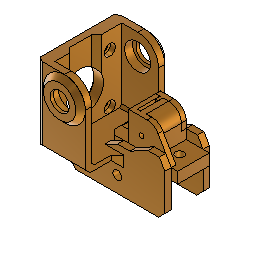
Worm Gear Buddy 0.8M Wide (Autodesk Fusion 360 design; units mm, degrees)
description: Worm Gear Drive bracket
part number: Worm Gear Buddy
Autodesk Fusion 360 part; units mm, degrees
note: some values were not read from the file. Chosen so that the rebuilt part matches the saved one: which face or edge a step refers to. Set by a fixed rule: which sketch regions a step uses; the direction of a hole.
sketch "Sketch2" plane through (0, 0, 0) normal (1, 0, 0) x (0, 1, 0)
  line L0 (0, 0) -> (48.25, 0)
  line L1 (50, 20) -> (50, 73.5)
  line L2 (0, 73.5) -> (0, 0)
  circle A0 centre (23, 42) radius 11.5
  line L3 (23, 0) -> (23, 73.5) construction
  line L4 (4, 73.5) -> (4, 23)
  line L5 (46, 73.5) -> (46, 23)
  line L6 (0, 20) -> (50, 20)
  line L7 (4, 23) -> (46, 23)
  line L8 (24.25, 20) -> (24.25, 0)
  line L9 (20.25, 20) -> (20.25, 0)
  line L10 (38.5, 26.5) -> (7.5, 26.5) construction
  line L11 (7.5, 26.5) -> (7.5, 57.5) construction
  line L12 (7.5, 57.5) -> (38.5, 57.5) construction
  line L13 (38.5, 57.5) -> (38.5, 26.5) construction
  line L14 (38.5, 26.5) -> (7.5, 57.5) construction
  line L15 (7.5, 26.5) -> (38.5, 57.5) construction
  line L16 (44.25, 20) -> (44.25, 0)
  line L17 (0, 73.5) -> (50, 73.5)
  line L18 (4, 20) -> (4, 0)
  circle A1 centre (7.5, 57.5) radius 3.5 construction
  line L19 (48.25, 20) -> (48.25, 0)
  dimension "d2076" = 0
  dimension "d2077" = 0
  dimension "d2078" = 0
  dimension "d2079" = 0
  dimension "d2092" = 0
  dimension "d2093" = 0
  dimension "d2094" = 0
  dimension "d2095" = 0
  dimension "d2312" = 0
  dimension "d2313" = 0
  dimension "d2314" = 0
  dimension "d2315" = 0
  dimension "d2324" = 0
  dimension "d2325" = 0
  dimension "d2326" = 0
  dimension "d2327" = 0
  dimension "d2544" = 0
  dimension "d2545" = 0
  dimension "d2546" = 0
  dimension "d2547" = 0
  dimension "d2572" = 0
  dimension "d2573" = 0
  dimension "d2574" = 0
  dimension "d2575" = 0
  dimension "d2728" = 0
  dimension "d2729" = 0
  dimension "d2730" = 0
  dimension "d2731" = 0
  dimension "d2896" = 0
  dimension "d2897" = 0
  dimension "d2898" = 0
  dimension "d2899" = 0
  dimension "d2949" = 0
  dimension "d2950" = 0
  dimension "d2951" = 0
  dimension "d2952" = 0
  dimension "d2957" = 0
  dimension "d2958" = 0
  dimension "d2959" = 0
  dimension "d2960" = 0
  dimension "d2961" = 0
  dimension "d2962" = 0
  dimension "d2963" = 0
  dimension "d2964" = 0
  dimension "d3029" = 0
  dimension "d3030" = 0
  dimension "d3031" = 0
  dimension "d3032" = 0
  dimension "d3037" = 0
  dimension "d3038" = 0
  dimension "d3039" = 0
  dimension "d3040" = 0
  dimension "d3045" = 0
  dimension "d3046" = 0
  dimension "d3047" = 0
  dimension "d3048" = 0
  dimension "d12_1" = 23
  dimension "d43" = 0
  dimension "d44" = 0
  dimension "d45" = 0
  dimension "d46" = 0
  dimension "d65" = 0
  dimension "d66" = 0
  dimension "d67" = 0
  dimension "d68" = 0
  dimension "d81" = 0
  dimension "d82" = 0
  dimension "d83" = 0
  dimension "d84" = 0
  dimension "d103" = 31.5
  dimension "d106" = 4
  dimension "d137" = 0
  dimension "d138" = 0
  dimension "d139" = 0
  dimension "d140" = 0
  dimension "d145" = 0
  dimension "d146" = 0
  dimension "d147" = 0
  dimension "d148" = 0
  dimension "d153" = 0
  dimension "d154" = 0
  dimension "d155" = 0
  dimension "d156" = 0
  dimension "d160" = 20
  dimension "d164" = 23
  dimension "d174" = 0
  dimension "d175" = 0
  dimension "d176" = 0
  dimension "d177" = 0
  dimension "d182" = 0
  dimension "d183" = 0
  dimension "d184" = 0
  dimension "d185" = 0
  dimension "d194" = 0
  dimension "d195" = 0
  dimension "d196" = 0
  dimension "d197" = 0
  dimension "d202" = 0
  dimension "d203" = 0
  dimension "d204" = 0
  dimension "d205" = 0
  dimension "d220" = 0
  dimension "d221" = 0
  dimension "d222" = 0
  dimension "d223" = 0
  dimension "d228" = 0
  dimension "d229" = 0
  dimension "d230" = 0
  dimension "d231" = 0
  dimension "d250" = 0
  dimension "d251" = 0
  dimension "d252" = 0
  dimension "d253" = 0
  dimension "d264" = 0
  dimension "d265" = 0
  dimension "d266" = 0
  dimension "d267" = 0
  dimension "d272" = 0
  dimension "d273" = 0
  dimension "d274" = 0
  dimension "d275" = 0
  dimension "d304" = 0
  dimension "d305" = 0
  dimension "d306" = 0
  dimension "d307" = 0
  dimension "d316" = 0
  dimension "d317" = 0
  dimension "d318" = 0
  dimension "d319" = 0
  dimension "d328" = 0
  dimension "d329" = 0
  dimension "d330" = 0
  dimension "d331" = 0
  dimension "d336" = 0
  dimension "d337" = 0
  dimension "d338" = 0
  dimension "d339" = 0
  dimension "d376" = 0
  dimension "d377" = 0
  dimension "d378" = 0
  dimension "d379" = 0
  dimension "d398" = 0
  dimension "d399" = 0
  dimension "d400" = 0
  dimension "d401" = 0
  dimension "d406" = 0
  dimension "d407" = 0
  dimension "d408" = 0
  dimension "d409" = 0
  dimension "d414" = 0
  dimension "d415" = 0
  dimension "d416" = 0
  dimension "d417" = 0
  dimension "d434" = 0
  dimension "d435" = 0
  dimension "d436" = 0
  dimension "d437" = 0
  dimension "d450" = 0
  dimension "d451" = 0
  dimension "d452" = 0
  dimension "d453" = 0
  dimension "d482" = 0
  dimension "d483" = 0
  dimension "d484" = 0
  dimension "d485" = 0
  dimension "d490" = 0
  dimension "d491" = 0
  dimension "d492" = 0
  dimension "d493" = 0
  dimension "d498" = 0
  dimension "d499" = 0
  dimension "d500" = 0
  dimension "d501" = 0
  dimension "d518" = 0
  dimension "d519" = 0
  dimension "d520" = 0
  dimension "d521" = 0
  dimension "d538" = 0
  dimension "d539" = 0
  dimension "d540" = 0
  dimension "d541" = 0
  dimension "d546" = 0
  dimension "d547" = 0
  dimension "d548" = 0
  dimension "d549" = 0
  dimension "d554" = 0
  dimension "d555" = 0
  dimension "d556" = 0
  dimension "d557" = 0
  dimension "d562" = 0
  dimension "d563" = 0
  dimension "d564" = 0
  dimension "d565" = 0
  dimension "d575" = 0
  dimension "d576" = 0
  dimension "d577" = 0
  dimension "d578" = 0
  dimension "d583" = 0
  dimension "d584" = 0
  dimension "d585" = 0
  dimension "d586" = 0
  dimension "d629" = 0
  dimension "d630" = 0
  dimension "d631" = 0
  dimension "d632" = 0
  dimension "d637" = 0
  dimension "d638" = 0
  dimension "d639" = 0
  dimension "d640" = 0
  dimension "d645" = 0
  dimension "d646" = 0
  dimension "d647" = 0
  dimension "d648" = 0
  dimension "d705" = 4
  dimension "d706" = 31
  dimension "d707" = 31
  dimension "d708" = 3
  dimension "d716" = 22
  dimension "d735" = 0
  dimension "d736" = 0
  dimension "d737" = 0
  dimension "d738" = 0
  dimension "d743" = 0
  dimension "d744" = 0
  dimension "d745" = 0
  dimension "d746" = 0
  dimension "d751" = 0
  dimension "d752" = 0
  dimension "d753" = 0
  dimension "d754" = 0
  dimension "d759" = 0
  dimension "d760" = 0
  dimension "d761" = 0
  dimension "d762" = 0
  dimension "d825" = 0
  dimension "d826" = 0
  dimension "d827" = 0
  dimension "d828" = 0
  dimension "d833" = 0
  dimension "d834" = 0
  dimension "d835" = 0
  dimension "d836" = 0
  dimension "d841" = 0
  dimension "d842" = 0
  dimension "d843" = 0
  dimension "d844" = 0
  dimension "d849" = 0
  dimension "d850" = 0
  dimension "d851" = 0
  dimension "d852" = 0
  dimension "d868" = 19
  dimension "d869" = 4
  dimension "d870" = 20
  dimension "d871" = 4
  dimension "d872" = 4
  dimension "d873" = 7
  dimension "d879" = 0
  dimension "d880" = 0
  dimension "d881" = 0
  dimension "d882" = 0
  dimension "d884" = 1.75
  dimension "d897" = 0
  dimension "d898" = 0
  dimension "d899" = 0
  dimension "d900" = 0
  dimension "d916" = 0
  dimension "d917" = 0
  dimension "d918" = 0
  dimension "d919" = 0
  dimension "d929" = 0
  dimension "d930" = 0
  dimension "d931" = 0
  dimension "d932" = 0
  dimension "d957" = 0
  dimension "d958" = 0
  dimension "d959" = 0
  dimension "d960" = 0
  dimension "d973" = 0
  dimension "d974" = 0
  dimension "d975" = 0
  dimension "d976" = 0
  dimension "d985" = 0
  dimension "d986" = 0
  dimension "d987" = 0
  dimension "d988" = 0
  dimension "d1013" = 0
  dimension "d1014" = 0
  dimension "d1015" = 0
  dimension "d1016" = 0
  dimension "d1021" = 0
  dimension "d1022" = 0
  dimension "d1023" = 0
  dimension "d1024" = 0
  dimension "d1029" = 0
  dimension "d1030" = 0
  dimension "d1031" = 0
  dimension "d1032" = 0
  dimension "d1037" = 0
  dimension "d1038" = 0
  dimension "d1039" = 0
  dimension "d1040" = 0
  measures "d12_1" diameter of A0
  measures "d706" distance of L0.start
  measures "d868" distance of L0.start
  measures "d872" distance of L0.start
  measures "d873" diameter of A1
extrude "Extrude1" add sketch "Sketch2" along normal blind 7 contours L1 L2 L4 L5 L6 L7 L17 | L4 L5 L7 L17 makes body 1
sketch "Sketch10" plane through (7, 0, 0) normal (1, 0, 0) x (0, 1, 0)
  line L0 (-7, 73.65) -> (7, 73.65)
  line L1 (7, 73.65) -> (7, 0)
  line L2 (7, 0) -> (-7, 0)
  line L3 (-7, 0) -> (-7, 73.65)
  circle A0 centre (23, 42) radius 11.5
  line L4 (50, 73.5) -> (0, 73.5)
  line L5 (0, 20) -> (50, 20)
  line L6 (50, 20) -> (50, 73.5)
  line L7 (0, 73.5) -> (0, 20)
  dimension "d243" = 14
extrude "Extrude2" add sketch "Sketch2" along normal blind 30.125 contours L1 L2 L4 L5 L6 L7 L17 | L0 L6 L8 L9 | L0 L6 L16 L19 bodies 1
sketch "Sketch12" plane through (0, 0, 0) normal (0, -1, 0) x (1, 0, 0)
  line L0 (17, 42) -> (17, 72.65) construction
  circle A0 centre (17, 55.2) radius 8.125
  line L1 (7, 42) -> (17, 42) construction
  circle A1 centre (17, 55.2) radius 6
  circle A2 centre (17, 55.2) radius 13.125
  line L2 (0, 20) -> (27.25, 20)
  line L3 (7, 53.5) -> (7, 30.5)
  line L4 (0, 53.5) -> (0, 30.5)
  line L5 (30.125, 73.5) -> (0, 73.5)
  line L6 (0, 20) -> (30.125, 20)
  dimension "d166" = 16.25
  dimension "d167" = 13.2
  dimension "d207" = 12
  dimension "d522" = 5
  dimension "d715" = 26.5
  dimension "d717" = 10
  dimension "d722" = 22
  measures "d166" diameter of A0
  measures "d207" diameter of A1
  measures "d522" distance of A0 A2
  measures "d722" distance of origin
extrude "Extrude17" cut sketch "Sketch12" against normal blind 60 contours A0 | A1 bodies 1
extrude "Extrude21" add sketch "Sketch12" along normal blind 3 contours A0 | A2 bodies 1
extrude "Extrude49" [suppressed]
move_face "OffsetFaces10" offset -1 1 faces at (24.3641, 0, 54.4983) on bodies 1
chamfer "Chamfer26" distance 3 angle 45 1 edges at (4.7632, -3, 50.4538) on bodies 1
sketch "Sketch15" plane through (0, 50, 0) normal (0, 1, 0) x (-1, 0, 0)
  line L0 (0, 20) -> (0, 73.5)
  line L1 (-30.125, 73.5) -> (-30.125, 20)
  circle A0 centre (-17, 55.2) radius 8.125
  circle A1 centre (-17, 55.2) radius 13.125
  line L2 (0, 73.5) -> (-30.125, 73.5)
  line L3 (-30.125, 20) -> (0, 20)
  circle A2 centre (-17, 55.2) radius 8.125
  circle A3 centre (-17, 55.2) radius 6
  dimension "d807" = 16.25
  dimension "d808" = 5
  measures "d807" diameter of A0
  measures "d808" distance of A0 A1
extrude "Extrude29" add sketch "Sketch15" along normal blind 3 contours A1 | A0 A2 bodies 1
move_face "OffsetFaces11" offset -1 1 faces at (24.3641, 50, 54.4983) on bodies 1
chamfer "Chamfer27" distance 3 angle 45 1 edges at (29.2368, 53, 50.4538) on bodies 1
hole "Hole2" at (0, 38.5, 57.5) at (0, 7.5, 57.5) at (0, 7.5, 26.5) at (0, 38.5, 26.5) direction (1, 0, 0) diameter 3.4 depth 30 tip angle 118 bodies 1
sketch "Sketch16" plane through (7, 0, 0) normal (1, 0, 0) x (0, 1, 0)
  circle A0 centre (7.5, 26.5) radius 1.7
  circle A1 centre (38.5, 57.5) radius 1.7
  circle A2 centre (38.5, 26.5) radius 1.7
  line L0 (4, 23) -> (46, 23)
  line L1 (46, 23) -> (46, 73.5)
  circle A3 centre (23, 42) radius 11.5
  line L2 (16, 73.5) -> (30, 73.5)
  line L3 (30, 73.5) -> (30, 36.5233)
  line L4 (30, 36.5233) -> (16, 36.5233)
  line L5 (16, 36.5233) -> (16, 73.5)
  circle A4 centre (38.5, 57.5) radius 3.5
  circle A5 centre (7.5, 57.5) radius 3.5
  circle A6 centre (7.5, 26.5) radius 3.5
  circle A7 centre (38.5, 26.5) radius 3.5
  line L6 (46, 73.5) -> (4, 73.5)
  line L7 (4, 73.5) -> (4, 23)
  circle A8 centre (7.5, 57.5) radius 1.7
  line L8 (23, 42) -> (23, 36.5233)
  dimension "d810" = 14
  dimension "d814" = 7
  dimension "d816" = 360
  measures "d810" distance of origin
  measures "d814" diameter of A4
extrude "Extrude30" cut sketch "Sketch16" against normal blind 3 contours A7 | A5 | A6 | A3 L2 L3 L5 L6 | A4 bodies 1
chamfer "Chamfer28" distance 3 angle 45 2 edges at (7, 30, 62.3121) (7, 16, 62.3121) on bodies 1
chamfer "Chamfer32" distance 1 angle 45 1 edges at (0, 12.2782, 46.1586) on bodies 1
chamfer "Chamfer57" distance 3 distance2 1.75 2 edges at (0, 50, 46.75) (0, 0, 46.75) measured on face at (15.3814, 50, 27.3706) measured on face at (15.3814, 0, 27.3706) on bodies 1
sketch "Sketch17" plane through (30.125, 0, 0) normal (1, 0, 0) x (0, 1, 0)
  line L0 (50, 20) -> (50, 55.2)
  line L1 (46, 73.5) -> (46, 23)
  line L2 (46, 23) -> (4, 23)
  line L3 (4, 23) -> (4, 73.5)
  line L4 (0, 73.5) -> (0, 55.2)
  line L5 (0, 20) -> (20.25, 20)
  line L6 (20.25, 20) -> (20.25, 0)
  line L7 (20.25, 0) -> (24.25, 0)
  line L8 (24.25, 0) -> (24.25, 20)
  line L9 (24.25, 20) -> (44.25, 20)
  line L10 (44.25, 20) -> (44.25, 0)
  line L11 (44.25, 0) -> (48.25, 0)
  line L12 (48.25, 0) -> (48.25, 20)
  line L13 (48.25, 20) -> (50, 20)
  line L14 (20.25, 20) -> (20.25, 23)
  line L15 (46, 23) -> (48.25, 23)
  line L16 (48.25, 20) -> (48.25, 23)
  line L17 (34.25, 20) -> (34.25, 68.3665)
  line L18 (50, 55.2) -> (50, 73.5)
  line L19 (50, 73.5) -> (46, 73.5)
  line L20 (4, 73.5) -> (0, 73.5)
  line L21 (0, 55.2) -> (0, 20)
extrude "Extrude32" add sketch "Sketch17" along normal blind 29.75 contours L2 L9 L10 L11 L12 L15 L16 L17 | L2 L6 L7 L8 L9 L14 L17 bodies 1
sketch "Sketch18" plane through (0, 44.25, 0) normal (0, -1, 0) x (1, 0, 0)
  line L0 (0, 20) -> (0, 0)
  line L1 (0, 0) -> (55, 0)
  line L2 (0, 0) -> (0, 20)
  line L3 (55, 0) -> (0, 0)
  line L4 (13, 10) -> (49.875, 10) construction
  line L5 (0, 20) -> (0, 0)
  line L6 (0, 0) -> (59.875, 0)
  line L7 (59.875, 23) -> (59.875, 0)
  line L8 (0, 20) -> (0, 0)
  dimension "d1228" = 10
  dimension "d1229" = 13
  measures "d1228" distance of L7
hole "Hole5" at (49.875, 44.25, 10) at (13, 44.25, 10) direction (0, 1, 0) diameter 5.5 depth 11 tip angle 118 bodies 1
hole "Hole6" at (29.9375, 24.25, 10) direction (0, -1, 0) diameter 5.5 depth 12 tip angle 118 bodies 1
sketch "Sketch22" plane through (0, 48.25, 0) normal (0, 1, 0) x (-1, 0, 0)
  line L0 (-59.875, 23) -> (-59.875, 0)
  line L1 (-30.125, 73.5) -> (-30.125, 55.2)
  line L2 (0, 20) -> (0, 0)
  circle A0 centre (-17, 55.2) radius 6
  line L3 (-3, 73.5) -> (-30.125, 73.5)
  line L4 (0, 0) -> (-59.875, 0)
  line L5 (-30.125, 23) -> (-59.875, 23)
  line L6 (-59.875, 23) -> (-59.875, 45.3923)
  line L7 (-59.875, 45.3923) -> (-33.125, 45.3923)
  line L8 (-33.125, 45.3923) -> (-33.125, 23)
  line L9 (-30.125, 20) -> (-30.125, 55.2)
  line L10 (-59.875, 23) -> (-41.25, 23)
  circle A1 centre (-17, 60.4) radius 6
  line L11 (-23, 55.2) -> (-23, 98.6748) construction
  line L12 (-23, 98.6748) -> (-23.75, 98.6748) construction
  line L13 (-23.75, 98.6748) -> (-23.75, 77.2864) construction
  circle A2 centre (-29.75, 90.4) radius 6 construction
  line L14 (-35.75, 90.4) -> (-35.75, 23.8063)
  line L15 (-35.75, 23.8063) -> (-37.75, 23.8063) construction
  line L16 (-37.75, 23.8063) -> (-37.75, 112.2143) construction
  circle A3 centre (-41.25, 35) radius 3.5
  circle A4 centre (-41.25, 35) radius 5.5
  arc A5 (-42.0357, 40.4436) -> (-37.75, 45.3923) centre (-42.75, 45.3923) ccw
  line L17 (-37.75, 45.3923) -> (-37.75, 57.1035) construction
  line L18 (-49.25, 45.3923) -> (-49.25, 27)
  line L19 (-49.25, 27) -> (-59.875, 27)
  circle A6 centre (-41.25, 35) radius 1.5
  line L20 (-33.125, 45.3923) -> (-30.125, 45.3923)
  line L21 (-49.25, 45.3923) -> (-59.875, 27)
  line L22 (-3, 73.5) -> (0, 73.5)
  line L23 (0, 73.5) -> (0, 20)
  line L24 (-30.125, 55.2) -> (-30.125, 23)
  dimension "d1262" = 3
  dimension "d1264" = 12
  dimension "d1265" = 0.75
  dimension "d1266" = 12
  dimension "d1267" = 2
  dimension "d1268" = 7
  dimension "d1269" = 2
  dimension "d1270" = 5
  dimension "d1272" = 4
  dimension "d1286" = 3
  dimension "d1287" = 2
  dimension "d1333" = 1.5
  dimension "d1334" = 2.5
  dimension "d1335" = 6.5
  dimension "d1336" = 2.5
  dimension "d1488" = 26.75
  dimension "d1489" = 30
  dimension "d1490" = 24.25
  measures "d1264" diameter of A1
  measures "d1266" diameter of A2
  measures "d1268" diameter of A3
  measures "d1269" distance of L14 L17
  measures "d1270" radius of A5
  measures "d1286" diameter of A6
  measures "d1287" distance of A3 A6
  measures "d1489" distance of L2.end
  measures "d1490" distance of L2.end
sketch "Sketch25" plane through (0, 0, 23) normal (0, 0, 1) x (-1, 0, 0)
  line L0 (-7, -7.5) -> (-7, -4)
  line L1 (-7, -4) -> (-30.125, -4)
  line L2 (-30.125, -4) -> (-30.125, -20.25)
  line L3 (-30.125, -20.25) -> (-59.875, -20.25)
  line L4 (-59.875, -20.25) -> (-59.875, -48.25)
  line L5 (-59.875, -48.25) -> (-30.125, -48.25)
  line L6 (-30.125, -48.25) -> (-30.125, -46)
  line L7 (-30.125, -46) -> (-7, -46)
  line L8 (-7, -46) -> (-7, -38.5)
  line L9 (-7, -38.5) -> (-7, -7.5)
  line L10 (0, -44.25) -> (-59.875, -44.25)
  line L11 (-59.875, -24.25) -> (0, -24.25)
  line L12 (-30.125, -48.25) -> (-30.125, -20.25)
extrude "Extrude42" add sketch "Sketch25" along normal blind 10 contours L3 L4 L11 L12 | L4 L5 L6 L10 L12 bodies 1
extrude "Extrude35" add sketch "Sketch22" against normal blind 14 from surface at -7 separate body contours L5 L6 L7 L8 L10 L14 A4 A5 L18 L19 | A3 makes body 2 at (37.7674, 31.9167, 34.6515) makes body 3 at (42.0417, 36.5833, 23)
extrude "Extrude36" add sketch "Sketch22" against normal blind 3 from surface at -21 contours L5 L6 L7 L8 L10 L14 A4 A5 L18 L19 | L18 L19 L21 | L7 L14 A4 A5 | A4 | A3 bodies 2 3
sketch "Sketch23" plane through (0, 41.25, 0) normal (0, 1, 0) x (1, 0, 0)
  line L0 (49.25, -45.3923) -> (49.25, -27)
  line L1 (49.25, -27) -> (59.875, -27)
  line L2 (59.875, -27) -> (59.875, -23)
  line L3 (59.875, -23) -> (33.125, -23)
  line L4 (33.125, -23) -> (33.125, -45.3923)
  line L5 (33.125, -45.3923) -> (35.75, -45.3923)
  line L6 (35.75, -45.3923) -> (35.75, -35)
  arc A0 (42.0357, -40.4436) -> (35.75, -35) centre (41.25, -35) ccw
  arc A1 (42.0357, -40.4436) -> (37.75, -45.3923) centre (42.75, -45.3923) ccw
  line L7 (37.75, -45.3923) -> (49.25, -45.3923)
  line L8 (49.25, -45.3923) -> (49.25, -23)
  line L9 (49.25, -45.3923) -> (33.125, -45.3923)
  circle A2 centre (41.25, -35) radius 3.5
  line L10 (59.875, -33) -> (30.125, -33)
  circle A3 centre (49.875, -10) radius 2.75
  circle A4 centre (13, -10) radius 2.75
  line L11 (0, 0) -> (0, -20)
  line L12 (0, -20) -> (30.125, -20)
  line L13 (30.125, -20) -> (30.125, -33)
  line L14 (30.125, -33) -> (59.875, -33) construction
  line L15 (59.875, -33) -> (59.875, 0)
  line L16 (59.875, 0) -> (0, 0)
  line L17 (30.125, -33) -> (59.875, -33)
  line L18 (30.125, -23) -> (59.875, -23)
  line L19 (59.875, -23) -> (59.875, -33)
  line L20 (59.875, -33) -> (30.125, -33)
  circle A5 centre (41.25, -35) radius 8.125
  line L21 (30.125, -33) -> (30.125, -23)
  circle A6 centre (41.25, -35) radius 1.5
  line L22 (49.25, -45.3923) -> (59.875, -27)
  line L23 (49.25, -33) -> (37.8688, -27)
  line L24 (49.25, -27) -> (30.125, -27)
extrude "Extrude44" add sketch "Sketch23" along normal blind 3 contours L0 L8 A5 L23 L24 | L1 L2 L3 L8 L15 L18 L19 | L3 L4 L8 L18 A5 L24 | A5 L23 L24 | A5 L24 | A5 L23 L24 bodies 2
sketch "Sketch26" plane through (33.125, 0, 0) normal (-1, 0, 0) x (0, -1, 0)
  line L0 (-41.25, 33) -> (-44.25, 33)
  line L1 (-44.25, 27) -> (-44.25, 23)
  line L2 (-44.25, 33) -> (-44.25, 27)
  line L3 (-41.25, 45.3923) -> (-41.25, 33)
  line L4 (-41.25, 45.3923) -> (-27.25, 45.3923)
  line L5 (-24.25, 23) -> (-24.25, 27)
  line L6 (-24.25, 23) -> (-44.25, 23)
  line L7 (-27.25, 45.3923) -> (-24.25, 45.3923)
  line L8 (-24.25, 27) -> (-24.25, 45.3923)
  line L9 (-44.25, 27) -> (-24.25, 27)
extrude "Extrude48" add sketch "Sketch26" along normal blind 12 contours L1 L5 L6 L9 bodies 2
chamfer "Chamfer58" distance 3 angle 45 2 edges at (21.125, 44.25, 25) (21.125, 24.25, 25) on bodies 2
hole "Hole7" at (55.25, 34.25, 20) direction (0, 0, 1) diameter 5.2 depth 21 tip angle 118 bodies 1 2
sketch "Sketch27" plane through (0, 0, 20) normal (0, 0, -1) x (1, 0, 0)
  circle A0 centre (55.25, -34.25) radius 2.6
  line L0 (59.875, -24.25) -> (59.875, -44.25)
  line L1 (55.25, -31.65) -> (59.875, -31.65)
  line L2 (59.875, -36.85) -> (55.25, -36.85)
extrude "Extrude50" cut sketch "Sketch27" against normal blind 7 contours A0 L0 L1 L2 bodies 1
hole "Hole8" at (27.125, 34.25, 20) direction (0, 0, 1) diameter 5.2 depth 12 tip angle 118 bodies 1 2
extrude "Extrude45" cut sketch "Sketch23" along normal mid plane 90 contours L10 L17 L20 A5 L23 | L10 L15 L17 L19 L20 L22 | A0 L10 L17 L20 A5 L23 | A0 A2 L10 L17 L20 | A0 L10 L17 L20 A5 L23 | A2 L10 L17 L20 | L4 L10 L17 L20 A5 L23 L24 | L4 L10 L13 L17 L20 L21 L24 picked at (41.4, -32.2528) bodies 1
chamfer "Chamfer53" distance 8 distance2 4 2 edges at (30.125, 22.25, 23) (30.125, 45.125, 23) measured on face at (13.0307, 26.2096, 23) measured on face at (13.0307, 26.2096, 23) on bodies 1
extrude "Extrude46" add sketch "Sketch23" along normal blind 3 and the other way blind 3 separate body contours A0 A2 L10 L17 L20 | L6 A0 A1 A2 L10 L17 L20 A5 | L6 A1 L9 A5 makes body 4
move_face "OffsetFaces12" offset -0.1 1 faces at (36.0482, 42.25, 33.2135) on bodies 4
move_face "OffsetFaces13" offset -0.1 1 faces at (38.9534, 42.25, 32.3589) on bodies 4
extrude "Extrude47" add sketch "Sketch23" along normal blind 3 contours L0 L8 L10 L17 L20 A5 | L10 L17 L20 A5 L23 | L0 A0 A1 L8 L10 L17 L20 A5 | A0 L10 L17 L20 A5 L23 | L0 A1 L7 L8 L9 A5 | A0 A2 L10 L17 L20 | L6 A0 A1 A2 L10 L17 L20 A5 | A0 L10 L17 L20 A5 L23 | L6 A1 L9 A5 | A2 L10 L17 L20 | A2 L10 L17 L20 | L6 A0 L10 L17 L20 A5 | L4 L10 L17 L20 A5 L23 L24 | L4 L5 L6 L9 A5 | L4 L10 L17 L20 A5 bodies 4
move_face "OffsetFaces15" offset -0.2 1 faces at (42.6595, 43.25, 35.513) on bodies 4
chamfer "Chamfer37" distance 4 angle 45 6 edges at (0, 22.25, 0) (0, 46.25, 0) (15.0625, 20.25, 20) (59.875, 22.25, 0) (59.875, 46.25, 0) (30.125, 20.25, 21.5) on bodies 1
chamfer "Chamfer38" distance 3 angle 45 1 edges at (16.5625, 0, 20) on bodies 1
chamfer "Chamfer51" distance 1.5 angle 45 2 edges at (18.5625, 4, 23) (14.5625, 46, 23) on bodies 1
chamfer "Chamfer54" distance 1.75 angle 45 2 edges at (15.0625, 48.25, 20) (30.125, 48.25, 23.5) on bodies 1
fillet "Fillet6" radius 8 3 edges at (49.25, 34.25, 45.3923) (49.25, 25.75, 45.3923) (49.25, 42.75, 45.3923) on bodies 2 4
chamfer "Chamfer56" distance 1 angle 45 1 edges at (39.665, 44.25, 34.3853) on bodies 4
move_face "OffsetFaces16" offset -5 1 faces at (4.6667, 42.4165, 73.5) on bodies 1
fillet "Fillet7" radius 13 2 edges at (30.125, 48, 68.5) (30.125, 2, 68.5) on bodies 1
copy_body "Body->Comp1" bodies 2 removing the originals makes body 5 in component "Z Belt Anchor M"
sketch "Sketch1" plane through (0, 0, 27) normal (0, 0, 1) x (-1, 0, 0) in component "Z Belt Anchor M"
  circle A0 centre (-27.125, -34.25) radius 2.6
  circle A1 centre (-55.25, -34.25) radius 2.6
  line L0 (-21.125, -27.25) -> (-24.125, -24.25)
  line L1 (-21.125, -41.25) -> (-21.125, -27.25)
  line L2 (-24.125, -44.25) -> (-21.125, -41.25)
  line L3 (-59.875, -44.25) -> (-24.125, -44.25)
  line L4 (-59.875, -24.25) -> (-59.875, -44.25)
  line L5 (-59.875, -24.25) -> (-24.125, -24.25)
  line L6 (-27.125, -36.85) -> (-21.125, -36.85)
  line L7 (-21.125, -31.65) -> (-27.125, -31.65)
  line L8 (-21.625, -36.85) -> (-21.625, -31.65)
  dimension "d1574" = 0.5
  measures "d1574" distance of L1 L8
extrude "Extrude1'" cut sketch "Sketch1" against normal blind 15 contours A0 | A0 L6 L7 L8 bodies 5 in component "Z Belt Anchor M"
sketch "Sketch2 (2)" plane through (0, 0, 27) normal (0, 0, 1) x (-1, 0, 0) in component "Z Belt Anchor M"
  line L0 (-59.875, -27.25) -> (-59.875, -44.25)
  line L1 (-59.875, -27.25) -> (-59.875, -24.25)
  circle A0 centre (-55.25, -34.25) radius 2.6
  line L2 (-49.25, -44.25) -> (-49.25, -27.25)
  line L3 (-49.25, -27.25) -> (-59.875, -27.25)
  line L4 (-59.875, -27.25) -> (-59.875, -44.25)
  line L5 (-59.875, -44.25) -> (-49.25, -44.25)
  line L6 (-59.875, -44.25) -> (-63.875, -44.25)
  line L7 (-63.875, -44.25) -> (-63.875, -24.25)
  line L8 (-63.875, -24.25) -> (-59.875, -24.25)
  line L9 (-59.875, -24.25) -> (-59.875, -44.25)
  dimension "d1582" = 4
extrude "Extrude2'" add sketch "Sketch2 (2)" against normal blind 7 contours L0 L1 L4 L6 L7 L8 L9 bodies 5 in component "Z Belt Anchor M"
copy_body "Body->Comp3" bodies 4 removing the originals makes body 6 in component "Z Belt Lock M"
component "Z Belt Anchor M" placed x (1, 0, 0) y (0, 1, 0) z (0, 0, 1) at (0, 0, 0)
component "Z Belt Lock M" placed x (1, 0, 0) y (0, 1, 0) z (0, 0, 1) at (0, 0, 0)
equation "d10_1 = 7 mm + 10 mm + ( 26.25 / 2 ) * 1 mm"
equation "d705 = d159"
equation "d807 = d166"
equation "d808 = d522"
equation "d869 = d705"
equation "d871 = d106"
equation "d872 = d869"
equation "d159 = d106"
named bodies: "Worm Gear Buddy", "Z Belt Anchor M", "Z Belt Lock M", "Worm Gear Buddy (1)", "Worm Gear Buddy (2)"
